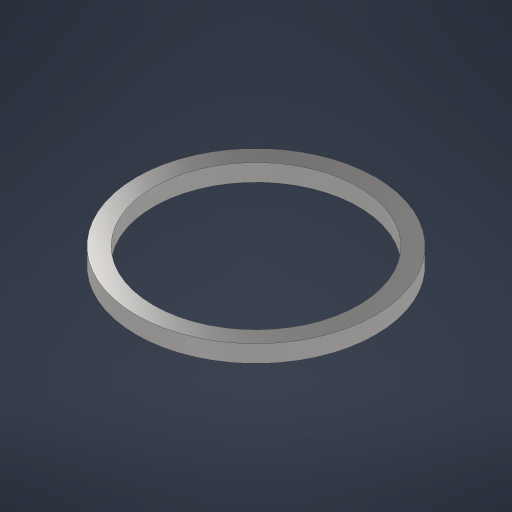
# Autodesk Inventor part: BEARING_HGB
Saved by Autodesk Inventor 2024.2 (Build 282272000, 272)
## iProperties
Created: 2026-01-16
Part Number: BEARING_HGB
Material: Stainless Steel
Document SubType Name: Modeling
Designer: 4aida
Density: 8 g/cm^3
Appearance: Semi-Polished
Author: 4aida
Autodesk Inventor part; units mm, degrees
ref_plane "YZ Plane" through (0, 0, 0) normal (1, 0, 0) x (0, 1, 0)
ref_plane "XZ Plane" through (0, 0, 0) normal (0, 1, 0) x (-1, 0, 0)
ref_plane "XY Plane" through (0, 0, 0) normal (0, 0, 1) x (1, 0, 0)
sketch "Sketch1" plane through (0, 0, 0) normal (1, 0, 0) x (0, 1, 0)
  line L0 (-3.175, 38.1) -> (3.175, 38.1)
  line L1 (3.175, 38.1) -> (3.175, 44.45)
  line L2 (3.175, 44.45) -> (-3.175, 44.45)
  line L3 (-3.175, 44.45) -> (-3.175, 38.1)
  line L4 (-3.175, 38.1) -> (3.175, 44.45) construction
  line L5 (3.175, 38.1) -> (-3.175, 44.45) construction
  line L6 (10.9322, 0) -> (-10.9322, 0)
  point P0 (0, 0)
  point P1 (0, 41.275)
  point P2 (0, 0)
  dimension "d0" = 76.2
  dimension "d1" = 88.9
  dimension "d2" = 6.35
  constraints: 14 end point, 3 midpoint, 2 horizontal, 2 parallel, 1 coincident, 1 perpendicular, 1 vertical alignment
  measures "d0" diameter of L0 L6
  measures "d1" diameter of L2 L6
  measures "d2" distance of L1.end L2.end
revolve "Revolution1" add sketch "Sketch1" angle 360 about axis through (0, 10.9322, 0) along (0, -1, 0)
body "Solid1"
